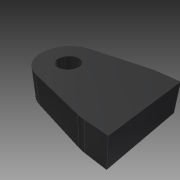
# Autodesk Inventor part: y_axis_cap_front_panel
Saved by Autodesk Inventor 2014 (Build 180170000, 170)
## iProperties
Created: 2014-01-23
Part Number: y_axis_cap_front_panel
Material: Generic
Document SubType Name: Modeling
Designer: buben
Density: 1 g/cm^3
Appearance: Anodized - Dark Gray
Author: buben
Autodesk Inventor part; units mm, degrees
ref_plane "YZ Plane" through (0, 0, 0) normal (1, 0, 0) x (0, 1, 0)
ref_plane "XZ Plane" through (0, 0, 0) normal (0, 1, 0) x (-1, 0, 0)
ref_plane "XY Plane" through (0, 0, 0) normal (0, 0, 1) x (1, 0, 0)
sketch "Sketch1" plane through (0, 0, 0) normal (0, 0, 1) x (1, 0, 0)
  line L0 (-1, 5.9161) -> (10.6667, 7.8881)
  arc A0 (12, 8) -> (10.6667, 7.8881) centre (12, 0) ccw
  line L1 (12, 8) -> (16, 8)
  line L2 (16, 8) -> (16, -8)
  line L3 (16, -8) -> (12, -8)
  arc A1 (10.6667, -7.8881) -> (12, -8) centre (12, 0) ccw
  line L4 (10.6667, -7.8881) -> (-1, -5.9161)
  arc A2 (-1, 5.9161) -> (-1, -5.9161) centre (0, 0) ccw
  circle A3 centre (0, 0) radius 2.25
  circle A4 centre (0, 0) radius 4.5 construction
  point P0 (16, 0)
  dimension "d0" = 8
  dimension "d1" = 8
  dimension "d2" = 6
  dimension "d3" = 4.5
  dimension "d4" = 9
  dimension "d5" = 12
  dimension "d6" = 4
  constraints: 10 end point, 6 point on circle, 5 centre point, 5 tangent, 4 coincident, 2 perpendicular, 1 horizontal, 1 horizontal alignment, 1 midpoint, 1 vertical alignment
  measures "d0" radius of A0
  measures "d1" radius of A1
  measures "d2" radius of A2
  measures "d3" diameter of A3
  measures "d4" diameter of A4
  measures "d5" distance of A0.centre point (0, 0)
  measures "d6" distance of L1.start L1.end
extrude "Extrusion1" add sketch "Sketch1" along normal blind 6
equation "\"d1\" = d0"
body "Solid1"
